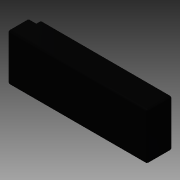
# Autodesk Inventor part: baterai
Saved by Autodesk Inventor 2015 (Build 190159000, 159)
## iProperties
Created: 2015-01-31
Part Number: baterai
Material: Generic
Document SubType Name: Modeling
Designer: Rafi Kurnia Putra
Density: 1 g/cm^3
Appearance: Anodized - Black
Author: Rafi Kurnia Putra
Autodesk Inventor part; units mm, degrees
ref_plane "YZ Plane" through (0, 0, 0) normal (1, 0, 0) x (0, 1, 0)
ref_plane "XZ Plane" through (0, 0, 0) normal (0, 1, 0) x (-1, 0, 0)
ref_plane "XY Plane" through (0, 0, 0) normal (0, 0, 1) x (1, 0, 0)
sketch "Sketch1" plane through (0, 0, 0) normal (0, 1, 0) x (-1, 0, 0)
  line L0 (69.21, 23.365) -> (-69.21, 23.365)
  line L1 (-69.21, 23.365) -> (-69.21, -23.365)
  line L2 (-69.21, -23.365) -> (69.21, -23.365)
  line L3 (69.21, -23.365) -> (69.21, 23.365)
  line L4 (69.21, 23.365) -> (-69.21, -23.365) construction
  line L5 (-69.21, 23.365) -> (69.21, -23.365) construction
  circle A0 centre (64.685, -18.84) radius 2
  circle A1 centre (64.685, 18.84) radius 2
  line L6 (69.21, -15) -> (62.845, -15)
  line L7 (60.845, -17) -> (60.845, -23.365)
  line L8 (69.21, 15) -> (62.845, 15)
  line L9 (60.845, 17) -> (60.845, 23.365)
  arc A2 (62.845, -15) -> (60.845, -17) centre (62.845, -17) ccw
  arc A3 (60.845, 17) -> (62.845, 15) centre (62.845, 17) ccw
  circle A4 centre (64.685, 0) radius 1
  point P0 (0, 0)
  point P1 (60.845, -15)
  point P2 (60.845, 15)
  dimension "d0" = 138.42
  dimension "d1" = 46.73
  dimension "d2" = 4
  dimension "d3" = 4
  dimension "d5" = 4.525
  dimension "d7" = 4.525
  dimension "d11" = 4.525
  dimension "d13" = 4.525
  dimension "d14" = 8.365
  dimension "d15" = 8.365
  dimension "d16" = 2
  dimension "d17" = 2
  dimension "d34" = 18.84
  constraints: 20 end point, 10 point on line, 5 centre point, 4 point on circle, 4 tangent, 3 perpendicular, 2 horizontal, 2 midpoint, 2 parallel, 1 equal radius, 1 vertical alignment
  measures "d0" distance of L2.end L1.end
  measures "d1" distance of L1.end L0.end
  measures "d2" diameter of A0
  measures "d3" diameter of A1
  measures "d5" distance from line of L3 A0.centre
  measures "d7" distance from line of L3 A1.centre
  measures "d11" distance from line of L2 A0.centre
  measures "d13" distance from line of L0 A1.centre
  measures "d14" distance of L6.start L2.end
  measures "d15" distance of L6.start point (60.845, -15)
  measures "d16" radius of A2
  measures "d17" diameter of A4
  measures "d34" distance of A4.centre A0.centre
extrude "Extrusion1" add sketch "Sketch1" along normal blind 25.3 contours L9 A3 L8 L3 L6 A2 L7 L2 L1 L0
extrude "Extrusion2" add sketch "Sketch1" along normal blind 20.2 contours L3 L8 A3 L9 L0 | L3 L2 L7 A2 L6
extrude "Extrusion3" add sketch "Sketch1" along normal blind 6 contours A0 | A1
extrude "Extrusion4" add sketch "Sketch1" along normal blind 11.1 contours A4
fillet "Fillet1" radius 2 18 edges at (0, 0, -23.365) (69.21, 0, 0) (0, 0, 23.365) (-69.21, 0, 0) (69.21, 12.65, 23.365) (69.21, 25.3, 0) (69.21, 12.65, -23.365) (4.1825, 25.3, -23.365) (-69.21, 10.1, -23.365) (-69.21, 10.1, 23.365) (4.1825, 25.3, 23.365) (-69.21, 25.3, 0) (-61.4308, 25.3, -15.5858) (-60.845, 25.3, -20.1825) (-66.0275, 25.3, -15) (-61.4308, 25.3, 15.5858) (-66.0275, 25.3, 15) (-60.845, 25.3, 20.1825)
fillet "Fillet2" radius 1 14 edges at (-68.6242, 20.2, -22.7792) (-64.0275, 20.2, -23.365) (-69.21, 20.2, -18.1825) (-60.845, 21.75, -23.365) (-60.2592, 24.7142, -22.7792) (-69.21, 21.75, -15) (-68.6242, 24.7142, -14.4142) (-68.6242, 20.2, 22.7792) (-64.0275, 20.2, 23.365) (-69.21, 20.2, 18.1825) (-68.6242, 24.7142, 14.4142) (-69.21, 21.75, 15) (-60.2592, 24.7142, 22.7792) (-60.845, 21.75, 23.365)
fillet "Fillet3" radius 0.25 10 edges at (-60.5521, 19.9071, 23.0721) (-61.4308, 20.2, 15.5858) (-65.5275, 20.2, 15) (-68.9171, 19.9071, 14.7071) (-60.845, 20.2, 19.6825) (-61.4308, 20.2, -15.5858) (-65.5275, 20.2, -15) (-68.9171, 19.9071, -14.7071) (-60.5521, 19.9071, -23.0721) (-60.845, 20.2, -19.6825)
fillet "Fillet4" radius 0.25 3 edges at (-62.685, 20.2, -18.84) (-63.685, 25.3, 0) (-62.685, 20.2, 18.84)
sketch "Sketch3" plane through (0, 25.3, 0) normal (0, 1, 0) x (1, 0, 0)
  line L0 (-54.5603, 15.2549) -> (-14.589, 15.2549) construction
  line L1 (-14.589, 15.2549) -> (-14.589, 8.9077) construction
  line L2 (-14.589, 8.9077) -> (-54.5603, 8.9077) construction
  line L3 (-54.5603, 8.9077) -> (-54.5603, 15.2549) construction
  line L4 (11.9565, 7.5587) -> (26.1762, 7.5587) construction
  line L5 (26.1762, 7.5587) -> (26.1762, 1.2474) construction
  line L6 (26.1762, 1.2474) -> (11.9565, 1.2474) construction
  line L7 (11.9565, 1.2474) -> (11.9565, 7.5587) construction
  point P0 (0, 0)
  dimension "d0" = 138.42
  constraints: 4 other
body "Solid1"
